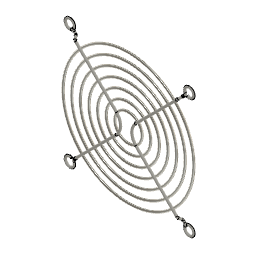
Fan guard (Autodesk Fusion 360 design; units mm, degrees)
Autodesk Fusion 360 part; units mm, degrees
note: some values were not read from the file. Chosen so that the rebuilt part matches the saved one: which face or edge a step refers to.
sketch "Sketch1" plane through (0, 0, 0) normal (0, 0, 1) x (1, 0, 0)
  circle A0 centre (12, 0) radius 1
  circle A1 centre (19.6, 0) radius 1
  circle A2 centre (27.2, 0) radius 1
  circle A3 centre (34.8, 0) radius 1
  circle A4 centre (42.4, 0) radius 1
  circle A5 centre (50, 0) radius 1
  circle A6 centre (57.6, 0) radius 1
  dimension "d1" = 2
  dimension "d2" = 2
  dimension "d3" = 2
  dimension "d4" = 2
  dimension "d5" = 2
  dimension "d6" = 2
  dimension "d7" = 2
  dimension "d8" = 12
  dimension "d9" = 7.6
  dimension "d10" = 7.6
  dimension "d11" = 7.6
  dimension "d12" = 7.6
  dimension "d13" = 7.6
  dimension "d14" = 7.6
  measures "d1" diameter of A0
  measures "d2" diameter of A1
  measures "d3" diameter of A2
  measures "d4" diameter of A3
  measures "d5" diameter of A4
  measures "d6" diameter of A5
  measures "d7" diameter of A6
  measures "d8" distance of origin A0.centre
  measures "d9" distance of A0.centre A1.centre
  measures "d10" distance of A1.centre A2.centre
  measures "d11" distance of A2.centre A3.centre
  measures "d12" distance of A3.centre A4.centre
  measures "d13" distance of A4.centre A5.centre
  measures "d14" distance of A5.centre A6.centre
revolve "Revolve1" add sketch "Sketch1" angle 360 about axis through (0, 1.75, 0) along (0, 1, 0) makes body 1 at (-37.0296, -0.0872, -22.6283) makes body 2 at (12.6831, -0.342, -2.564) makes body 3 at (-9.6849, -0.2849, -34.4221) makes body 4 at (20.9736, 0.0996, 46.4823) makes body 5 at (20.4779, 0.1981, -2.0491) makes body 6 at (25.9621, -0.2245, 10.9439) makes body 7 at (34.2034, -0.1161, 47.5741)
sketch "Sketch3" plane through (0, 0, 0) normal (0, 1, 0) x (1, 0, 0)
  line L0 (8.4853, -8.4853) -> (44.5477, -44.5477)
  line L1 (0, 0) -> (60, 0) construction
  line L2 (0, 0) -> (60, 0) construction
  arc A0 (4.9706, 0) -> (8.4853, -8.4853) centre (16.9706, 0) ccw
  dimension "d16" = 45
  dimension "d17" = 63
  dimension "d20" = 12
  constraint horizontal L1
  constraint coincident L1.start L2.start
  constraint horizontal L2
  constraint tangent L0 A0
  constraint coincident L1 A0.start
  measures "d16" angle of L0 L1
  measures "d17" distance of L1.start L0.end
  measures "d20" radius of A0
ref_plane "WorkPlane1" through (26.5165, 0, 26.5165) normal (-0.707107, 0, 0.707107) x (0.707107, 0, 0.707107)
sketch "Sketch5" plane through (25.4558, 0, 25.4558) normal (-0.707107, 0, 0.707107) x (0.707107, 0, 0.707107)
  line L0 (27.114, 0) -> (27.114, 4.5555) construction
  line L1 (27.114, 1.5) -> (33.4909, 1.5) construction
  circle A0 centre (27.114, 1.5) radius 1.5 construction
  circle A1 centre (31.3566, 1.5) radius 1.5 construction
  line L2 (28.1747, 0.4394) -> (30.2959, 2.5606)
  arc A2 (27.114, 0) -> (28.1747, 0.4394) centre (27.114, 1.5) ccw
  arc A3 (31.3566, 3) -> (30.2959, 2.5606) centre (31.3566, 1.5) ccw
  line L3 (38.56, 10) -> (38.56, -10) construction
  line L4 (32.9, 5) -> (32.9, -1.7699) construction
  line L5 (31.3566, 3) -> (32.9, 3)
  point P0 (24, 0)
  point P1 (27, 0)
  dimension "d28" = 1.5
  dimension "d29" = 3
  dimension "d30" = 3
  dimension "d31" = 4.2426
  dimension "d128" = 38.56
  dimension "d130" = 5.66
  dimension "d133" = 1.5434
  constraint coincident L0 L1.start
  constraint perpendicular L0 L1
  constraint coincident L1.start A0.centre
  constraint coincident L1 A1.centre
  constraint coincident A0 L2.start
  constraint coincident A1 L2.end
  constraint tangent A1 L2
  constraint tangent A0 L2
  constraint coincident A1 A3.start
  constraint horizontal L1
  constraint concentric A1 A3
  constraint vertical L3
  constraint coincident L4 L5.end
  constraint tangent A1 L5
  constraint perpendicular L4 L5
  measures "d28" distance of L1 P0
  measures "d29" diameter of A0
  measures "d30" diameter of A1
  measures "d31" distance of L1.start A1.centre
  measures "d128" distance of origin L3
  measures "d130" distance of L3 L4
  measures "d133" distance of A3.start L5.end
sketch "Sketch6" plane through (0, 0, 0) normal (0, 0, 1) x (1, 0, 0)
  circle A0 centre (4.97, 0) radius 1
  dimension "d33" = 2
  measures "d33" diameter of A0
ref_plane "WorkPlane3" through (0, 3, 0) normal (0, 1, 0) x (0, 0, 1)
ref_plane "WorkPlane4" through (0, 3, 0) normal (0, 1, 0) x (0, 0, 1)
sketch "Sketch12" plane through (0, 3, 0) normal (0, 1, 0) x (1, 0, 0)
  line L0 (48.5806, -48.5806) -> (57.0257, -57.0257) construction
  line L1 (48.5806, -48.5806) -> (51.0806, -48.5806) construction
  line L2 (48.1622, -50.9906) -> (55.0484, -57.8768) construction
  line L3 (48.5806, -48.5806) -> (46.1513, -51.0099) construction
  line L4 (52.5806, -52.5806) -> (51.2446, -49.3552) construction
  line L5 (52.5806, -52.5806) -> (59.1856, -52.5806) construction
  arc A0 (48.9711, -50.8567) -> (51.0499, -48.8851) centre (52.5806, -52.5806) ccw
  arc A1 (48.9711, -50.8567) -> (48.5806, -48.5806) centre (47.1664, -49.9948) ccw
  line L6 (52.5, 0) -> (52.5, -65) construction
  line L7 (40, -52.5) -> (65, -52.5) construction
  point P0 (47.6283, -47.6283)
  dimension "d100" = 45
  dimension "d103" = 2
  dimension "d104" = 8
  dimension "d105" = 112.5
  dimension "d125" = 52.5
  dimension "d126" = 52.5
  dimension "d132" = 5.6569
  constraint horizontal L1
  constraint parallel L0 L2
  constraint perpendicular L2 L3
  constraint coincident L2 A1.centre
  constraint coincident L3 A1.centre
  constraint coincident L0 L4.start
  constraint tangent A0 A1
  constraint horizontal L5
  constraint coincident L4.start L5.start
  constraint coincident L4 A0.end
  constraint vertical L6
  constraint horizontal L7
  measures "d100" angle of L0 L1
  measures "d103" distance of L0 L2
  measures "d104" diameter of A0
  measures "d105" angle of L4 L5
  measures "d125" distance of origin L6
  measures "d126" distance of origin L7
  measures "d132" distance of L0.start L4.start
sweep "Sweep6" add profiles "Sketch6" path "Sketch3" along A0 L0 section 1 separate body makes body 8
sweep "Sweep8" add 1 faces at (44.2955, -0.2606, 44.8) path "Sketch5" along A2 L2 A3 L5 on bodies 8 bodies 8
sweep "Sweep9" add 1 faces at (48.6606, 2.2962, 48.6175) path "Sketch12" along A0 A1 on bodies 8 bodies 8
mirror "Mirror3" about plane through (0, 0, 0) normal (0, 0, 1) of bodies 8 makes body 9
combine "Combine3" operation add target body 8 tool bodies 9
mirror "Mirror4" about plane through (0, 0, 0) normal (1, 0, 0) of bodies 8 makes body 10
move_body "Move3" bodies 8 10 to x (1, 0, 0) y (0, 1, 0) z (0, 0, 1) at (0, -2, 0)
equation "d2 = d1"
equation "d3 = d1"
equation "d4 = d1"
equation "d5 = d1"
equation "d6 = d1"
equation "d7 = d1"
equation "d10 = d9"
equation "d11 = d9"
equation "d12 = d9"
equation "d13 = d9"
equation "d14 = d9"
equation "d30 = d29"
equation "d31 = 2 * 0.7071 * d29"
equation "d125 = ( 105 / 2 ) * 1 mm"
equation "d126 = d125"
named bodies: "Ring 5", "Ring 1", "Ring 4", "Ring 6", "Ring 2", "Ring 3", "Ring 7", "Joiner 1", "Joiner 1 (1)", "Joiner 2"
